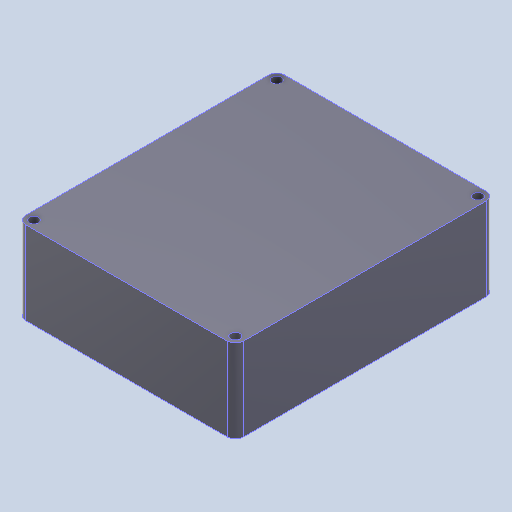
# Autodesk Inventor part: motor_driver
Saved by Autodesk Inventor 2025.3 (Build 293356030, 356C)
## iProperties
Created: 2025-08-30
Part Number: motor_driver
Material: ABS 플라스틱
Document SubType Name: Modeling
Designer: MSI
Density: 1.06 g/cm^3
Appearance: 매끄러움 - 흰색
Mass: 116.584 g
Surface Area: 204.009 cm^2
Volume: 109.985 cm^3
Author: MSI
Autodesk Inventor part; units mm, degrees
ref_plane "YZ Plane" through (0, 0, 0) normal (1, 0, 0) x (0, 1, 0)
ref_plane "XZ Plane" through (0, 0, 0) normal (0, 1, 0) x (-1, 0, 0)
ref_plane "XY Plane" through (0, 0, 0) normal (0, 0, 1) x (1, 0, 0)
sketch "스케치1" plane through (0, 0, 0) normal (0, 1, 0) x (-1, 0, 0)
  line L0 (39.37, -46.84) -> (-39.37, -46.84)
  line L1 (-39.37, -46.84) -> (-39.37, 46.84)
  line L2 (-39.37, 46.84) -> (39.37, 46.84)
  line L3 (39.37, 46.84) -> (39.37, -46.84)
  line L4 (39.37, -46.84) -> (-39.37, 46.84) construction
  line L5 (-39.37, -46.84) -> (39.37, 46.84) construction
  point P0 (0, 0)
  dimension "d0" = 78.74
  dimension "d1" = 93.68
  constraints: 12 end point, 2 midpoint, 2 parallel, 1 horizontal, 1 perpendicular
  measures "d0" distance of L1.end L2.end
  measures "d1" distance of L0.end L1.end
extrude "돌출1" add sketch "스케치1" along normal blind 30
fillet "모깎기1" radius 3 4 edges at (39.37, 15, 46.84) (39.37, 15, -46.84) (-39.37, 15, -46.84) (-39.37, 15, 46.84)
sketch "스케치2" plane through (0, 30, 0) normal (0, 1, 0) x (1, 0, 0)
  arc A0 (36.37, -46.84) -> (39.37, -43.84) centre (36.37, -43.84) ccw projected
  arc A1 (39.37, 43.84) -> (36.37, 46.84) centre (36.37, 43.84) ccw projected
  arc A2 (-36.37, 46.84) -> (-39.37, 43.84) centre (-36.37, 43.84) ccw projected
  arc A3 (-39.37, -43.84) -> (-36.37, -46.84) centre (-36.37, -43.84) ccw projected
  point P0 (0, 0)
  constraints: 4 coincident
hole "구멍1" at (36.37, 30, 43.84) at (36.37, 30, -43.84) at (-36.37, 30, -43.84) at (-36.37, 30, 43.84) direction (0, -1, 0) diameter 3.4 end through all clearance for "Countersunk Flat Head Screw ISO 2009/7046" size "M3" standard "ISO"
